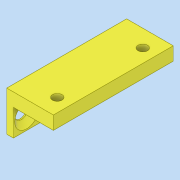
# Autodesk Inventor part: limitSwitchHolderMount
Saved by Autodesk Inventor 2017 (Build 210142000, 142)
## iProperties
Created: 2016-12-04
Part Number: limitSwitchHolderMount
Material: ABS Plastic
Document SubType Name: Modeling
Designer: techn
Density: 1.06 g/cm^3
Appearance: Smooth - Yellow
Author: techn
Autodesk Inventor part; units mm, degrees
ref_plane "YZ Plane" through (0, 0, 0) normal (1, 0, 0) x (0, 1, 0)
ref_plane "XZ Plane" through (0, 0, 0) normal (0, 1, 0) x (-1, 0, 0)
ref_plane "XY Plane" through (0, 0, 0) normal (0, 0, 1) x (1, 0, 0)
sketch "Sketch1" plane through (0, 0, 0) normal (0, 1, 0) x (-1, 0, 0)
  line L0 (0, 0) -> (9.525, 0)
  line L1 (9.525, 0) -> (9.525, -28.575)
  line L2 (9.525, -28.575) -> (0, -28.575)
  line L3 (0, -28.575) -> (0, 0)
  circle A0 centre (3.175, -4.0894) radius 1.143
  circle A1 centre (3.175, -24.4856) radius 1.143
  dimension "d0" = 9.525
  dimension "d1" = 28.575
  dimension "d2" = 2.286
  dimension "d3" = 2.286
  dimension "d4" = 20.3962
  dimension "d5" = 4.0894
  dimension "d6" = 6.35
  constraints: 8 end point, 2 centre point, 2 parallel, 1 horizontal, 1 perpendicular
  measures "d0" distance of L1.end L2.end
  measures "d1" distance of L0.end L1.end
  measures "d2" diameter of A0
  measures "d3" diameter of A1
  measures "d4" distance of A1.centre A0.centre
  measures "d5" distance from line of L2 A1.centre
  measures "d6" distance from line of L1 A1.centre
extrude "Extrusion1" add sketch "Sketch1" along normal blind 3.175
sketch "Sketch2" plane through (-9.525, 0, -28.575) normal (-1, 0, 0) x (0, 0, 1)
  line L0 (28.575, 0) -> (0, 0) projected
  line L1 (28.575, 0) -> (28.575, 3.175) projected
  line L2 (0, 3.175) -> (28.575, 3.175) projected
  line L3 (0, 0) -> (0, 3.175) projected
  line L4 (28.575, 3.175) -> (0, 3.175) projected
  line L5 (28.575, 3.175) -> (0, 3.175)
  line L6 (0, 3.175) -> (0, -6.35)
  line L7 (0, -6.35) -> (28.575, -6.35)
  line L8 (28.575, -6.35) -> (28.575, 3.175)
  dimension "d9" = 9.525
  constraints: 8 end point, 2 parallel, 1 horizontal, 1 perpendicular
  measures "d9" distance of L6.end L5.end
extrude "Extrusion2" add sketch "Sketch2" along normal blind 1.5875
sketch "Sketch3" plane through (-9.525, 0, -28.575) normal (1, 0, 0) x (0, 0, -1)
  line L0 (-28.575, 0) -> (0, 0) projected
  line L1 (-28.575, -6.35) -> (-28.575, 0) projected
  line L2 (0, -6.35) -> (-28.575, -6.35) projected
  line L3 (0, 0) -> (0, -6.35) projected
  circle A0 centre (-25.4, -3.175) radius 1.5875
  circle A1 centre (-3.175, -3.175) radius 1.5875
  point P0 (-28.575, 0)
  dimension "d12" = 3.175
  dimension "d13" = 3.175
  dimension "d14" = 3.175
  dimension "d15" = 3.175
  constraints: 2 centre point
  measures "d12" diameter of A0
  measures "d13" diameter of A1
  measures "d14" distance from line of L1 A0.centre
  measures "d15" distance from line of L3 A1.centre
extrude "Extrusion3" cut sketch "Sketch3" against normal blind 1.5875 contours A0 | A1
chamfer "Chamfer1" distance 1.27 angle 45 2 edges at (-9.525, -3.175, -1.5875) (-9.525, -3.175, -23.8125)
body "Solid1"
